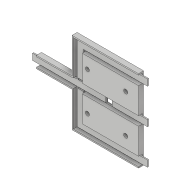
# Autodesk Inventor part: bottomv6
Saved by Autodesk Inventor 2019 (Build 230136000, 136)
## iProperties
Created: 2020-08-26
Part Number: bottomv6
Material: Generic
Document SubType Name: Modeling
Designer: UCLA
Density: 1 g/cm^3
Appearance: Default
Author: UCLA
Autodesk Inventor part; units mm, degrees
ref_plane "YZ Plane" through (0, 0, 0) normal (1, 0, 0) x (0, 1, 0)
ref_plane "XZ Plane" through (0, 0, 0) normal (0, 1, 0) x (-1, 0, 0)
ref_plane "XY Plane" through (0, 0, 0) normal (0, 0, 1) x (1, 0, 0)
sketch "Sketch2" plane through (0, 0, 0) normal (0, 0, 1) x (1, 0, 0)
  line L0 (0, 2.45) -> (0, -2.45)
  line L1 (0, 2.45) -> (30, 2.45)
  line L2 (30, 2.45) -> (30, 29.95)
  line L3 (30, 29.95) -> (80, 29.95)
  line L4 (80, 29.95) -> (80, 25.05)
  line L5 (34.9, 3.55) -> (30.85, 3.55)
  line L6 (30.85, 3.55) -> (30.85, 2.45)
  line L7 (30.85, 2.45) -> (80, 2.45)
  line L8 (80, 2.45) -> (80, -2.45)
  line L9 (80, -2.45) -> (30.85, -2.45)
  line L10 (30.85, -2.45) -> (30.85, -3.55)
  line L11 (30.85, -3.55) -> (34.9, -3.55)
  line L12 (34.9, -3.55) -> (34.9, -25.05)
  line L13 (34.9, 3.55) -> (34.9, 25.05)
  line L14 (80, 25.05) -> (34.9, 25.05)
  line L15 (0, -2.45) -> (30, -2.45)
  line L16 (30, -2.45) -> (30, -29.95)
  line L17 (80, -25.05) -> (80, -29.95)
  line L18 (80, -29.95) -> (30, -29.95)
  line L19 (80, -25.05) -> (34.9, -25.05)
  line L20 (0, 2.45) -> (0, 3.55)
  line L21 (0, 3.55) -> (28.9, 3.55)
  line L22 (28.9, 3.55) -> (28.9, 31.05)
  line L23 (80, 29.95) -> (80, 31.05)
  line L24 (80, 31.05) -> (28.9, 31.05)
  line L25 (80, 25.05) -> (80, 23.95)
  line L26 (80, 23.95) -> (36, 23.95)
  line L27 (80, 2.45) -> (80, 3.55)
  line L28 (80, 3.55) -> (36, 3.55)
  line L29 (36, 3.55) -> (36, 23.95)
  line L30 (0, -2.45) -> (0, -3.55)
  line L31 (0, -3.55) -> (28.9, -3.55)
  line L32 (28.9, -3.55) -> (28.9, -31.05)
  line L33 (80, -2.45) -> (80, -3.55)
  line L34 (80, -3.55) -> (36, -3.55)
  line L35 (36, -3.55) -> (36, -23.95)
  line L36 (80, -25.05) -> (80, -23.95)
  line L37 (80, -23.95) -> (36, -23.95)
  line L38 (80, -29.95) -> (80, -31.05)
  line L39 (80, -31.05) -> (28.9, -31.05)
  line L40 (0, 3.55) -> (0, 4.55)
  line L41 (0, 4.55) -> (27.9, 4.55)
  line L42 (27.9, 4.55) -> (27.9, 32.05)
  line L43 (80, 3.55) -> (80, 4.55)
  line L44 (80, 4.55) -> (37, 4.55)
  line L45 (37, 4.55) -> (37, 22.95)
  line L46 (80, 23.95) -> (80, 22.95)
  line L47 (80, 22.95) -> (37, 22.95)
  line L48 (80, 31.05) -> (80, 32.05)
  line L49 (80, 32.05) -> (27.9, 32.05)
  line L50 (0, -3.55) -> (0, -4.55)
  line L51 (0, -4.55) -> (27.9, -4.55)
  line L52 (27.9, -4.55) -> (27.9, -32.05)
  line L53 (80, -31.05) -> (80, -32.05)
  line L54 (80, -32.05) -> (27.9, -32.05)
  line L55 (80, -23.95) -> (80, -22.95)
  line L56 (80, -22.95) -> (37, -22.95)
  line L57 (80, -3.55) -> (80, -4.55)
  line L58 (80, -4.55) -> (37, -4.55)
  line L59 (37, -4.55) -> (37, -22.95)
  line L60 (80, 22.95) -> (80, 4.55)
  line L61 (80, -4.55) -> (80, -22.95)
  line L62 (40, -15) -> (70, -15) construction
  line L63 (70, -15) -> (70, 15) construction
  line L64 (70, 15) -> (40, 15) construction
  line L65 (40, 15) -> (40, -15) construction
  line L66 (40, -15) -> (70, 15) construction
  line L67 (70, -15) -> (40, 15) construction
  line L68 (55, 0) -> (0, 0) construction
  circle A0 centre (70, 15) radius 1.6
  circle A1 centre (40, 15) radius 1.6
  circle A2 centre (70, -15) radius 1.6
  circle A3 centre (40, -15) radius 1.6
  dimension "d21" = 4.9
  dimension "d23" = 4.9
  dimension "d27" = 30
  dimension "d28" = 4.05
  dimension "d29" = 1.1
  dimension "d31" = 1.1
  dimension "d33" = 1.1
  dimension "d34" = 1.1
  dimension "d35" = 1.1
  dimension "d36" = 1.1
  dimension "d37" = 1.1
  dimension "d38" = 1.1
  dimension "d39" = 1
  dimension "d40" = 1
  dimension "d41" = 1
  dimension "d42" = 1
  dimension "d43" = 1
  dimension "d44" = 1
  dimension "d54" = 30
  dimension "d55" = 30
  dimension "d57" = 3.2
  dimension "d58" = 3.2
  dimension "d59" = 3.2
  dimension "d60" = 3.2
  dimension "d75" = 1.1
  dimension "d76" = 1
  dimension "d77" = 1.1
  dimension "d78" = 1
  dimension "d79" = 4.9
  dimension "d80" = 4.9
  dimension "d81" = 50.1
  dimension "d83" = 55
  dimension "d84" = 80
  constraints: 138 end point, 31 perpendicular, 17 vertical, 16 collinear, 8 parallel, 7 horizontal, 5 coincident, 4 centre point, 3 midpoint, 1 point on line, 1 other
  measures "d21" distance of L0.start L0.end
  measures "d23" distance between parallel lines of L2 L13
  measures "d27" distance of L0.start L1.end
  measures "d28" distance between parallel lines of L13 L6
  measures "d29" distance between parallel lines of L7 L5
  measures "d31" distance between parallel lines of L9 L11
  measures "d33" distance of L0.start L20.end
  measures "d34" distance of L4.end L25.end
  measures "d35" distance of L17.start L36.end
  measures "d36" distance of L17.end L38.end
  measures "d37" distance between parallel lines of L24 L3
  measures "d38" distance between parallel lines of L15 L31
  measures "d39" distance of L20.end L40.end
  measures "d40" distance of L25.end L46.end
  measures "d41" distance of L23.end L48.end
  measures "d42" distance of L30.end L50.end
  measures "d43" distance of L38.end L53.end
  measures "d44" distance of L36.end L55.end
  measures "d54" distance of L64.end L63.end
  measures "d55" distance of L63.end L62.end
  measures "d57" diameter of A0
  measures "d58" diameter of A1
  measures "d59" diameter of A2
  measures "d60" diameter of A3
  measures "d75" distance between parallel lines of L2 L22
  measures "d76" distance between parallel lines of L22 L42
  measures "d77" distance between parallel lines of L29 L13
  measures "d78" distance between parallel lines of L45 L29
  measures "d79" distance between parallel lines of L14 L3
  measures "d80" distance between parallel lines of L18 L19
  measures "d81" distance between parallel lines of L19 L14
  measures "d83" distance from line of L68.start L0
  measures "d84" distance between parallel lines of L0 L60
extrude "Extrusion1" add sketch "Sketch2" along normal blind 2 contours L1 L2 L3 L4 L14 L13 L5 L6 L7 L8 L9 L10 L11 L12 L19 L17 L18 L16 L15 L0
extrude "Extrusion2" add sketch "Sketch2" along normal blind 1 contours L1 L2 L3 L4 L14 L13 L5 L6 L7 L8 L9 L10 L11 L12 L19 L17 L18 L16 L15 L0 | L20 L21 L22 L24 L23 L3 L2 L1 | L15 L16 L18 L38 L39 L32 L31 L30 | L25 L26 L29 L28 L27 L7 L6 L5 L13 L14 | L19 L12 L11 L10 L9 L33 L34 L35 L37 L36
extrude "Extrusion3" add sketch "Sketch2" along normal blind 4 contours L40 L41 L42 L49 L48 L24 L22 L21 | L31 L32 L39 L53 L54 L52 L51 L50 | L46 L47 L45 L44 L43 L28 L29 L26 | L37 L35 L34 L57 L58 L59 L56 L55
extrude "Extrusion4" add sketch "Sketch2" along normal up to surface (4 mm away) contours L60 L44 L45 L47 | L56 L59 L58 L61
sketch "Sketch3" plane through (0, 0, 0) normal (0, 0, -1) x (-1, 0, 0)
  line L0 (-52.5, -2.5) -> (-57.5, -2.5)
  line L1 (-57.5, -2.5) -> (-57.5, 2.5)
  line L2 (-57.5, 2.5) -> (-52.5, 2.5)
  line L3 (-52.5, 2.5) -> (-52.5, -2.5)
  line L4 (-52.5, -2.5) -> (-57.5, 2.5) construction
  line L5 (-57.5, -2.5) -> (-52.5, 2.5) construction
  line L6 (-55, 0) -> (0, 0) construction
  line L7 (-80, -4.55) -> (-80, 4.55) projected
  line L8 (-49, -6) -> (-61, -6)
  line L9 (-61, -6) -> (-61, 6)
  line L10 (-61, 6) -> (-49, 6)
  line L11 (-49, 6) -> (-49, -6)
  line L12 (-49, -6) -> (-61, 6) construction
  line L13 (-61, -6) -> (-49, 6) construction
  dimension "d51" = 5
  dimension "d52" = 5
  dimension "d53" = 25
  dimension "d65" = 12
  dimension "d66" = 12
  constraints: 26 end point, 4 midpoint, 4 parallel, 3 horizontal, 2 perpendicular
  measures "d51" distance of L1.end L2.end
  measures "d52" distance of L0.end L1.end
  measures "d53" distance from line of L7 L6.start
  measures "d65" distance of L9.end L10.end
  measures "d66" distance of L8.end L9.end
extrude "Extrusion5" cut sketch "Sketch3" against normal blind 2 contours L0 L1 L2 L3
extrude "Extrusion6" cut sketch "Sketch3" against normal blind 0.5
sketch "Sketch4" plane through (80, -2.45, 2) normal (1, 0, 0) x (0, 0, -1)
  line L0 (0, 27.5) -> (0, 32.4) projected
  line L1 (0, 32.4) -> (0.9, 32.4)
  line L2 (0.9, 32.4) -> (0.9, 27.5)
  line L3 (0.9, 27.5) -> (0, 27.5)
  line L4 (0, 27.5) -> (0, 32.4)
  line L5 (1, 27.5) -> (0, 27.5) projected
  line L6 (0, 0) -> (0, 4.9) projected
  line L7 (0, 4.9) -> (0.9, 4.9)
  line L8 (0.9, 4.9) -> (0.9, 0)
  line L9 (0.9, 0) -> (0, 0)
  line L10 (0, 0) -> (0, 4.9)
  line L11 (0.9, -22.6) -> (0, -22.6)
  line L12 (0.9, -22.6) -> (0.9, -27.5)
  line L13 (0.9, -27.5) -> (0, -27.5)
  line L14 (0, -27.5) -> (0, -22.6)
  line L15 (1, -27.5) -> (0, -27.5) projected
  line L16 (1, 0) -> (0, 0) projected
  line L17 (1, -22.6) -> (0, -22.6) projected
  line L18 (0, -27.5) -> (0, -22.6) projected
  point P0 (2, 2.45)
  dimension "d69" = 0.9
  constraints: 24 end point, 6 collinear, 5 parallel, 2 horizontal, 2 perpendicular, 1 point on line
  measures "d69" distance between parallel lines of L0 L2
extrude "Extrusion7" add sketch "Sketch4" along normal blind 5
sketch "Sketch5" plane through (0, -2.45, 2) normal (-1, 0, 0) x (0, 0, 1)
  line L0 (0, 4.9) -> (-0.9, 4.9)
  line L1 (-0.9, 4.9) -> (-0.9, 0)
  line L2 (-0.9, 0) -> (0, 0)
  line L3 (0, 0) -> (0, 4.9)
  line L4 (0, 4.9) -> (0, 0) projected
  line L5 (-1, 0) -> (0, 0) projected
  line L6 (-1, 4.9) -> (0, 4.9) projected
  line L7 (-1, 6) -> (-1, 4.9) projected
  point P0 (-2, 2.45)
  dimension "d72" = 0.1
  constraints: 8 end point, 3 collinear, 2 parallel, 1 horizontal, 1 perpendicular
  measures "d72" distance between parallel lines of L7 L1
extrude "Extrusion8" add sketch "Sketch5" along normal blind 5
body "Solid1"
